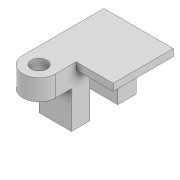
# Autodesk Inventor part: optical sensor
Saved by Autodesk Inventor 2022 (Build 260153000, 153)
## iProperties
Created: 2024-08-30
Part Number: optical sensor
Material: Generic
Document SubType Name: Modeling
Designer: david
Density: 1 g/cm^3
Appearance: Default
Author: david
Autodesk Inventor part; units mm, degrees
ref_plane "YZ Plane" through (0, 0, 0) normal (1, 0, 0) x (0, 1, 0)
ref_plane "XZ Plane" through (0, 0, 0) normal (0, 1, 0) x (-1, 0, 0)
ref_plane "XY Plane" through (0, 0, 0) normal (0, 0, 1) x (1, 0, 0)
sketch "Sketch1" plane through (0, 0, 0) normal (0, 1, 0) x (-1, 0, 0)
  line L0 (0, -6.5) -> (-15, -6.5)
  line L1 (-15, -6.5) -> (-15, 6.5)
  line L2 (-15, 6.5) -> (0, 6.5)
  line L3 (0, 6.5) -> (0, -6.5)
  line L4 (0, -6.5) -> (-15, 6.5) construction
  line L5 (-15, -6.5) -> (0, 6.5) construction
  line L6 (0, -20.3) -> (0, 20.3) projected
  line L7 (-3.5, -11) -> (-3.5, 11) construction
  line L8 (0, -11) -> (0, -6.5) construction
  line L9 (-7, 11) -> (-7, -6.5)
  arc A0 (-7, -11) -> (0, -11) centre (-3.5, -11) ccw construction
  arc A1 (0, 11) -> (-7, 11) centre (-3.5, 11) ccw
  line L10 (0, -6.5) -> (0, 11)
  line L11 (-7, -6.5) -> (-7, -11) construction
  point P0 (0, 0)
  point P1 (-7.5, 0)
  point P2 (-7.5, 0)
  point P3 (-3.5, 0)
  point P4 (0, 11)
  point P5 (-7, 6.5)
  point P6 (0, 6.5)
  dimension "d0" = 13
  dimension "d1" = 15
  dimension "d3" = 7
  dimension "d4" = 8
  dimension "d5" = 8
  constraints: 24 end point, 8 tangent, 7 parallel, 4 midpoint, 4 point on circle, 3 collinear, 2 centre point, 1 horizontal, 1 horizontal alignment, 1 perpendicular, 1 point on line
  measures "d0" distance of L2.end L0.start
  measures "d1" distance of L1.end L2.end
  measures "d3" diameter of A1
extrude "Extrusion1" add sketch "Sketch1" along normal blind 1.5
sketch "Sketch2" plane through (0, 0, 0) normal (0, -1, 0) x (1, 0, 0)
  line L0 (7, 11) -> (7, 6.5) projected
  arc A0 (7, 11) -> (0, 11) centre (3.5, 11) ccw projected
  line L1 (0, -6.5) -> (0, 11) projected
  line L2 (15, -6.5) -> (0, -6.5) projected
  line L3 (15, 6.5) -> (15, -6.5) projected
  line L4 (7, 6.5) -> (15, 6.5) projected
  line L5 (7, 11) -> (7, 6.5) projected
  line L6 (7, 6.5) -> (7, -6.5)
  point P0 (0, 0)
  constraints: 2 end point, 1 perpendicular, 1 point on line
extrude "Extrusion2" add sketch "Sketch2" along normal blind 3 contours L0 L6 L2 L1 A0
sketch "Sketch3" plane through (0, 1.5, -6.5) normal (-1, 0, 0) x (0, 0, 1)
  line L0 (14, -12.5) -> (10, -12.5)
  line L1 (10, -12.5) -> (10, -4.5)
  line L2 (10, -4.5) -> (14, -4.5)
  line L3 (14, -4.5) -> (14, -12.5)
  line L4 (17.5, -4.5) -> (0, -4.5) projected
  line L5 (13, -1.5) -> (13, 0) projected
  line L6 (0, -4.5) -> (4, -4.5)
  line L7 (4, -4.5) -> (4, -12.5)
  line L8 (4, -12.5) -> (0, -12.5)
  line L9 (0, -12.5) -> (0, -4.5)
  point P0 (6.5, -1.5)
  dimension "d10" = 4
  dimension "d11" = 8
  dimension "d12" = 1
  dimension "d13" = 4
  constraints: 16 end point, 4 parallel, 2 collinear, 2 horizontal, 2 perpendicular
  measures "d10" distance of L0.start L0.end
  measures "d11" distance between parallel lines of L4 L0
  measures "d12" distance between parallel lines of L5 L3
  measures "d13" distance of L7.end L8.end
extrude "Extrusion3" add sketch "Sketch3" against normal up to surface (7 mm away)
sketch "Sketch4" plane through (0, -3, 0) normal (0, -1, 0) x (1, 0, 0)
  arc A0 (7, 11) -> (0, 11) centre (3.5, 11) ccw projected
  point P0 (0, 0)
  constraints: 1 coincident
hole "Hole1" at (3.5, -3, 11) direction (0, 1, 0) diameter 3.4 end through all
equation "\"d5\" = d4"
equation "\"d13\" = d10"
body "Solid1"
